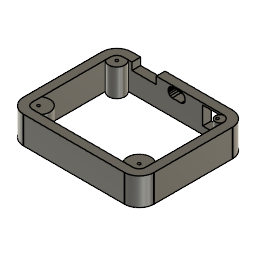
spelarö (Autodesk Fusion 360 design; units mm, degrees)
description: KiCad electronic assembly
part number: spelar_ 1
part number: KEY-SMD_6P-L10.2-W10.2-H10.0-LS11.7-P6.5
part number: C145910
part number: plate and holes
part number: circle001
part number: circle002
part number: circle003
part number: circle004
part number: border001
part number: border002
part number: ShapeString099
part number: ShapeString100
part number: ShapeString101
part number: ShapeString102
part number: ShapeString103
part number: ShapeString104
part number: silk_upper
part number: cupper_upper
part number: cupper_bottom
part number: mask_bottom
part number: res_silk
part number: res_silk001
part number: res_silk002
part number: res_silk003
part number: res_silk004
part number: res_silk005
part number: cap_silk_up
part number: cap_silk_dwn
part number: cap_silk001
part number: cap_silk_up001
part number: cap_silk_dwn001
part number: cap_silk002
part number: sot23_left
part number: sot23_right
part number: sot23_001
part number: sot23_left001
part number: sot23_right001
part number: sot23_002
part number: u2_silk002
part number: sd_silk001
part number: line_silk001
part number: line_silk002
part number: ShapeString067
part number: ShapeString105
part number: ShapeString106
part number: ShapeString107
part number: ShapeString108
part number: ShapeString109
part number: touch
part number: ShapeString068
part number: ShapeString110
part number: ShapeString111
part number: ShapeString112
part number: ShapeString113
part number: ShapeString114
part number: ShapeString069
part number: ShapeString115
part number: ShapeString116
part number: ShapeString117
part number: ShapeString118
part number: ShapeString070
part number: ShapeString119
part number: ShapeString120
part number: ShapeString121
part number: ShapeString122
part number: ShapeString123
part number: ShapeString071
part number: ShapeString124
part number: ShapeString125
part number: ShapeString126
part number: ShapeString127
part number: ShapeString073
part number: ShapeString128
part number: ShapeString129
part number: ShapeString130
part number: ShapeString131
part number: ShapeString132
part number: ShapeString072
part number: ShapeString133
part number: ShapeString134
part number: ShapeString135
part number: ShapeString136
part number: ShapeString137
part number: ShapeString138
part number: ShapeString139
part number: ShapeString140
part number: ShapeString141
part number: ShapeString074
part number: ShapeString142
part number: ShapeString143
part number: ShapeString144
part number: ShapeString075
part number: ShapeString145
part number: ShapeString146
part number: ShapeString147
part number: ShapeString076
part number: ShapeString148
part number: ShapeString149
part number: ShapeString150
part number: ShapeString151
part number: ShapeString152
part number: ShapeString153
part number: ShapeString154
part number: ShapeString155
part number: ShapeString156
part number: ShapeString077
part number: ShapeString157
part number: ShapeString158
part number: ShapeString078
part number: ShapeString159
part number: ShapeString160
part number: ShapeString161
part number: ShapeString162
part number: ShapeString163
part number: ShapeString079
part number: ShapeString164
part number: ShapeString165
part number: ShapeString080
part number: ShapeString166
part number: ShapeString167
part number: ShapeString168
part number: ShapeString081
part number: ShapeString169
part number: ShapeString170
part number: ShapeString171
part number: ShapeString082
part number: ShapeString172
part number: ShapeString173
part number: ShapeString174
part number: ShapeString175
part number: ShapeString176
part number: ShapeString177
part number: ShapeString083
part number: ShapeString178
part number: ShapeString179
part number: ShapeString180
part number: ShapeString181
part number: ShapeString182
part number: ShapeString183
part number: ShapeString184
part number: ShapeString084
part number: ShapeString185
part number: ShapeString186
part number: ShapeString187
part number: ShapeString188
part number: ShapeString189
part number: ShapeString190
part number: ShapeString191
part number: ShapeString085
part number: ShapeString192
part number: ShapeString193
part number: ShapeString194
part number: ShapeString195
part number: ShapeString196
part number: ShapeString086
part number: ShapeString197
part number: ShapeString198
part number: ShapeString199
part number: ShapeString200
part number: ShapeString201
part number: ShapeString202
part number: ShapeString203
part number: ShapeString204
part number: ShapeString205
part number: ShapeString206
part number: ShapeString207
part number: ShapeString208
part number: ShapeString209
part number: ShapeString210
part number: ShapeString211
part number: ShapeString212
part number: ShapeString213
part number: ShapeString214
part number: ShapeString215
part number: ShapeString216
part number: ShapeString217
part number: ShapeString218
part number: ShapeString219
part number: ShapeString220
part number: ShapeString221
part number: ShapeString222
part number: ShapeString087
part number: ShapeString223
part number: ShapeString224
part number: ShapeString088
part number: ShapeString225
part number: ShapeString226
part number: ShapeString089
part number: ShapeString227
part number: ShapeString228
part number: ShapeString090
part number: ShapeString229
part number: ShapeString230
part number: ShapeString091
part number: ShapeString231
part number: ShapeString232
part number: ShapeString092
part number: ShapeString233
part number: ShapeString234
part number: ShapeString093
part number: ShapeString235
part number: ShapeString236
part number: ShapeString094
part number: ShapeString237
part number: ShapeString238
part number: ShapeString095
part number: ShapeString239
part number: ShapeString240
part number: ShapeString096
part number: ShapeString241
part number: ShapeString242
part number: ShapeString097
part number: ShapeString243
part number: ShapeString244
part number: ShapeString098
part number: ShapeString245
part number: ShapeString246
part number: text
part number: j_silk006
part number: silk_bottom
part number: contact01
part number: contact02
part number: contact03
part number: contact04
part number: contact05
part number: contact06
part number: contact07
part number: contact08
part number: frame001
part number: contact09
part number: cover
part number: contact11
part number: contact10
part number: SD slot
part number: TSSOP16_001
part number: TSSOP16_002
part number: TSSOP16_003
part number: TSSOP16_004
part number: TSSOP16_005
part number: TSSOP16_006
part number: TSSOP16_007
part number: TSSOP16_008
part number: TSSOP16_009
part number: ShapeString066
part number: ShapeString247
part number: ShapeString248
part number: ShapeString249
part number: ShapeString250
part number: ShapeString251
part number: ShapeString252
part number: ShapeString253
part number: TSSOP16_010
part number: body
part number: contact1
part number: contact2
part number: label
part number: ShapeString001
part number: ShapeString254
part number: ShapeString255
part number: ShapeString256
part number: Part010
part number: SMD_resistor001
part number: body003
part number: contact016
part number: contact017
part number: label001
part number: ShapeString002
part number: ShapeString257
part number: ShapeString258
part number: ShapeString259
part number: Part013
part number: SMD_resistor002
part number: body004
part number: contact018
part number: contact019
part number: label002
part number: ShapeString003
part number: ShapeString260
part number: ShapeString261
part number: ShapeString262
part number: Part015
part number: SMD_resistor003
part number: body005
part number: contact020
part number: contact021
part number: label003
part number: ShapeString004
part number: ShapeString263
part number: ShapeString264
part number: ShapeString265
part number: Part017
part number: SMD_resistor004
part number: body006
part number: contact022
part number: contact023
part number: label004
part number: ShapeString005
part number: ShapeString266
part number: ShapeString267
part number: ShapeString268
part number: Part019
part number: SMD_resistor005
part number: body007
part number: contact024
part number: contact025
part number: label005
part number: ShapeString006
part number: ShapeString269
part number: ShapeString270
part number: ShapeString271
part number: Part021
part number: SMD_resistor006
part number: body008
part number: contact026
part number: contact027
part number: SMD_cap001
part number: body002
part number: contact014
part number: contact015
part number: SMD_cap002
part number: ShapeString064
part number: ShapeString272
part number: ShapeString273
part number: ShapeString274
part number: Pin036
part number: Pin035
part number: Pin1
part number: Case
part number: SOT23
part number: ShapeString065
part number: ShapeString275
part number: ShapeString276
part number: ShapeString277
part number: ShapeString278
part number: Pin039
part number: Pin038
part number: Pin037
part number: Case001
part number: SOT23-1
part number: parts
part number: Frame
part number: Pin01
part number: Pin002
part number: Pin003
part number: Pin004
part number: Pin005
part number: Pin006
part number: Pin007
part number: Pin008
part number: Pin009
part number: Pin010
part number: Pin011
part number: Pin012
part number: Pin013
part number: Pin014
part number: pls-14
part number: components
part number: mask_upper
part number: Board
part number: frame
part number: metal bandage
part number: light_shelf
part number: main_shelf
part number: tft_cable
part number: tft_matrix
part number: tft_board
part number: tft
part number: screen_film
part number: screen_glass
part number: screen
part number: Display
part number: touch_routs
part number: touch_protect
part number: touch_cable_contacts
part number: touch_cable_film
part number: touch_cable
part number: Touchscreen
part number: Display and Touchscreen
part number: 2.8''LCD_MSP2807
part number: LCD_MSP2807_fusion
part number: VS-1213-67-160GF
part number: C_1206_3216Metric
part number: TF-SMD_TF-012
part number: ESP32 S3 SUPERMINI
part number: ESP32-S3-ZERO
part number: FCR684205R ORJ5
part number: 4654_FCR684205T%20OTJ5
part number: spelarÃ¶_copper
part number: spelarÃ¶_pad
part number: spelarÃ¶_via
part number: spelarÃ¶_silkscreen
part number: spelarÃ¶_soldermask
part number: spelarÃ¶_PCB
Autodesk Fusion 360 part; units mm, degrees
(part 1 of 5)
sketch "Sketch1" plane through (0, 0, 1.56) normal (0, 0, 1) x (-1, 0, 0)
  arc A0 (-129.3118, 35.1924) -> (-124.5324, 39.9718) centre (-129.53, 40.19) ccw
  line L0 (-124.5324, 39.9718) -> (-124.53, 40.19)
  line L1 (-124.53, 40.19) -> (-124.53, 102.8)
  line L2 (-124.53, 102.8) -> (-124.5323, 103.0182)
  arc A1 (-124.5323, 103.0182) -> (-129.3118, 107.7977) centre (-129.53, 102.8) ccw
  line L3 (-129.3118, 107.7977) -> (-129.53, 107.8)
  line L4 (-129.53, 107.8) -> (-210.09, 107.8)
  line L5 (-210.09, 107.8) -> (-210.3082, 107.7977)
  arc A2 (-210.3082, 107.7977) -> (-215.0877, 103.0182) centre (-210.09, 102.8) ccw
  line L6 (-215.0877, 103.0182) -> (-215.09, 102.8)
  line L7 (-215.09, 102.8) -> (-215.09, 40.19)
  line L8 (-215.09, 40.19) -> (-215.0876, 39.9718)
  arc A3 (-215.0876, 39.9718) -> (-210.3082, 35.1924) centre (-210.09, 40.19) ccw
  line L9 (-210.3082, 35.1924) -> (-210.09, 35.19)
  line L10 (-210.09, 35.19) -> (-129.53, 35.19)
  line L11 (-129.53, 35.19) -> (-129.3118, 35.1924)
  circle A4 centre (-129.53, 102.8) radius 2.2
  circle A5 centre (-210.09, 102.8) radius 2.2
  line L12 (-153, 103.32) -> (-153, 104.72)
  line L13 (-153, 104.72) -> (-151, 104.72)
  line L14 (-151, 104.72) -> (-151, 103.32)
  line L15 (-151, 103.32) -> (-153, 103.32)
  line L16 (-164.46, 103.32) -> (-164.46, 104.72)
  line L17 (-164.46, 104.72) -> (-162.46, 104.72)
  line L18 (-162.46, 104.72) -> (-162.46, 103.32)
  line L19 (-162.46, 103.32) -> (-164.46, 103.32)
  circle A6 centre (-172, 103.08) radius 1.077
  circle A7 centre (-184.5, 103.08) radius 1.077
  line L20 (-153, 100.52) -> (-153, 101.92)
  line L21 (-153, 101.92) -> (-151, 101.92)
  line L22 (-151, 101.92) -> (-151, 100.52)
  line L23 (-151, 100.52) -> (-153, 100.52)
  line L24 (-164.46, 100.52) -> (-164.46, 101.92)
  line L25 (-164.46, 101.92) -> (-162.46, 101.92)
  line L26 (-162.46, 101.92) -> (-162.46, 100.52)
  line L27 (-162.46, 100.52) -> (-164.46, 100.52)
  arc A8 (-173.077, 97.105) -> (-172.975, 97.003) centre (-172.975, 97.105) ccw
  line L28 (-173.077, 97.105) -> (-173.077, 99.055)
  arc A9 (-172.975, 99.157) -> (-173.077, 99.055) centre (-172.975, 99.055) ccw
  line L29 (-172.975, 99.157) -> (-171.025, 99.157)
  arc A10 (-170.923, 99.055) -> (-171.025, 99.157) centre (-171.025, 99.055) ccw
  line L30 (-170.923, 99.055) -> (-170.923, 97.105)
  arc A11 (-171.025, 97.003) -> (-170.923, 97.105) centre (-171.025, 97.105) ccw
  line L31 (-171.025, 97.003) -> (-172.975, 97.003)
  circle A12 centre (-184.5, 98.08) radius 1.077
  line L32 (-153, 96.82) -> (-153, 98.22)
  line L33 (-153, 98.22) -> (-151, 98.22)
  line L34 (-151, 98.22) -> (-151, 96.82)
  line L35 (-151, 96.82) -> (-153, 96.82)
  line L36 (-164.46, 96.82) -> (-164.46, 98.22)
  line L37 (-164.46, 98.22) -> (-162.46, 98.22)
  line L38 (-162.46, 98.22) -> (-162.46, 96.82)
  line L39 (-162.46, 96.82) -> (-164.46, 96.82)
  line L40 (-212.43, 77.21) -> (-212.43, 78.91)
  line L41 (-212.43, 78.91) -> (-210.73, 78.91)
  line L42 (-210.73, 78.91) -> (-210.73, 77.21)
  line L43 (-210.73, 77.21) -> (-212.43, 77.21)
  circle A13 centre (-211.58, 75.52) radius 0.85
  circle A14 centre (-211.58, 72.98) radius 0.85
  circle A15 centre (-211.58, 70.44) radius 0.85
  circle A16 centre (-211.58, 67.9) radius 0.85
  circle A17 centre (-211.58, 65.36) radius 0.85
  circle A18 centre (-211.58, 62.82) radius 0.85
  circle A19 centre (-211.58, 60.28) radius 0.85
  circle A20 centre (-211.58, 57.74) radius 0.85
  circle A21 centre (-211.58, 55.2) radius 0.85
  circle A22 centre (-211.58, 52.66) radius 0.85
  circle A23 centre (-211.58, 50.12) radius 0.85
  circle A24 centre (-211.58, 47.58) radius 0.85
  circle A25 centre (-196.89, 46.1501) radius 0.6604
  circle A26 centre (-199.43, 46.1501) radius 0.6604
  circle A27 centre (-201.97, 46.1501) radius 0.6604
  circle A28 centre (-211.58, 45.04) radius 0.85
  circle A29 centre (-129.53, 40.19) radius 2.2
  circle A30 centre (-210.09, 40.19) radius 2.2
  arc A31 (-222.0862, 39.8056) -> (-210.4744, 28.1938) centre (-210.09, 40.19) ccw
  line L44 (-210.4744, 28.1938) -> (-210.1282, 28.19)
  line L45 (-210.1282, 28.19) -> (-129.4918, 28.19)
  line L46 (-129.4918, 28.19) -> (-129.1456, 28.1938)
  arc A32 (-129.1456, 28.1938) -> (-117.5338, 39.8056) centre (-129.53, 40.19) ccw
  line L47 (-117.5338, 39.8056) -> (-117.53, 40.1518)
  line L48 (-117.53, 40.1518) -> (-117.53, 102.8371)
  line L49 (-117.53, 102.8371) -> (-117.5337, 103.1831)
  arc A33 (-117.5337, 103.1831) -> (-129.1469, 114.7963) centre (-129.53, 102.8) ccw
  line L50 (-129.1469, 114.7963) -> (-129.4929, 114.8)
  line L51 (-129.4929, 114.8) -> (-210.1271, 114.8)
  line L52 (-210.1271, 114.8) -> (-210.4731, 114.7963)
  arc A34 (-210.4731, 114.7963) -> (-222.0863, 103.1831) centre (-210.09, 102.8) ccw
  line L53 (-222.0863, 103.1831) -> (-222.09, 102.8371)
  line L54 (-222.09, 102.8371) -> (-222.09, 40.1518)
  line L55 (-222.09, 40.1518) -> (-222.0862, 39.8056)
  dimension "d1" = 7
extrude "Extrude1" add sketch "Sketch1" against normal blind 22 contours A31 L44 L45 L46 A32 L47 L48 L49 A33 L50 L51 L52 A34 L53 L54 L55
sketch "Sketch2" plane through (0, -28.19, 0) normal (0, 1, 0) x (-1, 0, 0)
  line L0 (-129.4918, 1.56) -> (-210.1282, 1.56)
  line L1 (-210.1282, 1.56) -> (-210.1282, -20.44)
  line L2 (-210.1282, -20.44) -> (-129.4918, -20.44)
  line L3 (-129.4918, -20.44) -> (-129.4918, 1.56)
  line L4 (-153.8, -0.2) -> (-139, -0.2)
  line L5 (-139, -0.2) -> (-139, -2)
  line L6 (-139, -2) -> (-153.8, -2)
  line L7 (-153.8, -2) -> (-153.8, -0.2)
  line L8 (-156.1178, -4.3178) -> (-156.1178, 2.1178)
  line L9 (-156.1178, 2.1178) -> (-136.6822, 2.1178)
  line L10 (-136.6822, 2.1178) -> (-136.6822, -4.3178)
  line L11 (-136.6822, -4.3178) -> (-156.1178, -4.3178)
  dimension "d4" = -2.3178
  constraint horizontal L4
  constraint vertical L5
  constraint horizontal L6
  constraint vertical L7
extrude "Extrude2" cut sketch "Sketch2" against normal blind 7 contours L0 L8 L10 L11 | L4 L5 L6 L7
sketch "Sketch3" plane through (0, -28.19, 0) normal (0, 1, 0) x (-1, 0, 0)
  line L0 (-136.6822, 1.56) -> (-136.6822, -4.3178)
  line L1 (-136.6822, -4.3178) -> (-156.1178, -4.3178)
  line L2 (-156.1178, -4.3178) -> (-156.1178, 1.56)
  line L3 (-156.1178, 1.56) -> (-210.1282, 1.56)
  line L4 (-210.1282, 1.56) -> (-210.1282, -20.44)
  line L5 (-210.1282, -20.44) -> (-129.4918, -20.44)
  line L6 (-129.4918, -20.44) -> (-129.4918, 1.56)
  line L7 (-129.4918, 1.56) -> (-136.6822, 1.56)
  line L8 (-175.65, -1.85) -> (-169.25, -1.85)
  line L9 (-169.25, -1.85) -> (-168.6525, -2.0383)
  line L10 (-168.6525, -2.0383) -> (-168.3, -2.4)
  line L11 (-168.3, -2.4) -> (-168.1, -2.7)
  line L12 (-168.1, -2.7) -> (-168.0543, -2.9985)
  line L13 (-168.0543, -2.9985) -> (-168.0543, -3.7)
  line L14 (-168.0543, -3.7) -> (-168.1, -4.044)
  line L15 (-168.1, -4.044) -> (-168.2705, -4.3456)
  line L16 (-168.2705, -4.3456) -> (-168.5369, -4.6523)
  line L17 (-168.5369, -4.6523) -> (-169.2457, -4.8986)
  line L18 (-169.2457, -4.8986) -> (-175.7, -4.8986)
  line L19 (-175.7, -4.8986) -> (-176.2708, -4.724)
  line L20 (-176.2708, -4.724) -> (-176.6, -4.35)
  line L21 (-176.6, -4.35) -> (-176.8, -4)
  line L22 (-176.8, -4) -> (-176.85, -3.7)
  line L23 (-176.85, -3.7) -> (-176.8, -2.9)
  line L24 (-176.8, -2.9) -> (-176.6204, -2.414)
  line L25 (-176.6204, -2.414) -> (-176.1201, -1.9736)
  line L26 (-176.1201, -1.9736) -> (-175.65, -1.85)
  line L27 (-179.0982, -2.4144) -> (-178.5967, -1.0576)
  line L28 (-178.5967, -1.0576) -> (-177.2431, 0.1341)
  line L29 (-177.2431, 0.1341) -> (-175.9505, 0.474)
  line L30 (-175.9505, 0.474) -> (-168.8924, 0.474)
  line L31 (-168.8924, 0.474) -> (-167.3963, 0.0024)
  line L32 (-167.3963, 0.0024) -> (-166.4856, -0.9319)
  line L33 (-166.4856, -0.9319) -> (-165.8806, -1.8394)
  line L34 (-165.8806, -1.8394) -> (-165.7303, -2.8217)
  line L35 (-165.7303, -2.8217) -> (-165.7303, -3.8535)
  line L36 (-165.7303, -3.8535) -> (-165.8554, -4.7959)
  line L37 (-165.8554, -4.7959) -> (-166.3626, -5.6931)
  line L38 (-166.3626, -5.6931) -> (-167.1889, -6.6442)
  line L39 (-167.1889, -6.6442) -> (-168.8534, -7.2226)
  line L40 (-168.8534, -7.2226) -> (-176.0475, -7.2226)
  line L41 (-176.0475, -7.2226) -> (-177.5801, -6.7537)
  line L42 (-177.5801, -6.7537) -> (-178.5005, -5.7083)
  line L43 (-178.5005, -5.7083) -> (-179.0241, -4.7921)
  line L44 (-179.0241, -4.7921) -> (-179.1861, -3.8201)
  line L45 (-179.1861, -3.8201) -> (-179.0982, -2.4144)
  dimension "d7" = -2.324
  constraint horizontal L8
  constraint perpendicular L8 L13
  constraint parallel L8 L18
  constraint perpendicular L20 L25
extrude "Extrude3" cut sketch "Sketch3" against normal blind 7 contours L8 L9 L10 L11 L12 L13 L14 L15 L16 L17 L18 L19 L20 L21 L22 L23 L24 L25 L26 | L27 L28 L29 L30 L31 L32 L33 L34 L35 L36 L37 L38 L39 L40 L41 L42 L43 L44 L45
sketch "Sketch4" plane through (0, -28.19, 0) normal (0, 1, 0) x (-1, 0, 0)
  line L0 (-178.5005, -5.7083) -> (-179.0241, -4.7921)
  line L1 (-179.0241, -4.7921) -> (-179.1861, -3.8201)
  line L2 (-179.1861, -3.8201) -> (-179.0982, -2.4144)
  line L3 (-179.0982, -2.4144) -> (-178.5967, -1.0576)
  line L4 (-178.5967, -1.0576) -> (-177.2431, 0.1341)
  line L5 (-177.2431, 0.1341) -> (-175.9505, 0.474)
  line L6 (-175.9505, 0.474) -> (-168.8924, 0.474)
  line L7 (-168.8924, 0.474) -> (-167.3963, 0.0024)
  line L8 (-167.3963, 0.0024) -> (-166.4856, -0.9319)
  line L9 (-166.4856, -0.9319) -> (-165.8806, -1.8394)
  line L10 (-165.8806, -1.8394) -> (-165.7303, -2.8217)
  line L11 (-165.7303, -2.8217) -> (-165.7303, -3.8535)
  line L12 (-165.7303, -3.8535) -> (-165.8554, -4.7959)
  line L13 (-165.8554, -4.7959) -> (-166.3626, -5.6931)
  line L14 (-166.3626, -5.6931) -> (-167.1889, -6.6442)
  line L15 (-167.1889, -6.6442) -> (-168.8534, -7.2226)
  line L16 (-168.8534, -7.2226) -> (-176.0475, -7.2226)
  line L17 (-176.0475, -7.2226) -> (-177.5801, -6.7537)
  line L18 (-177.5801, -6.7537) -> (-178.5005, -5.7083)
  line L19 (-136.6822, 1.56) -> (-136.6822, -4.3178)
  line L20 (-136.6822, -4.3178) -> (-156.1178, -4.3178)
  line L21 (-156.1178, -4.3178) -> (-156.1178, 1.56)
  line L22 (-156.1178, 1.56) -> (-210.1282, 1.56)
  line L23 (-210.1282, 1.56) -> (-210.1282, -20.44)
  line L24 (-210.1282, -20.44) -> (-129.4918, -20.44)
  line L25 (-129.4918, -20.44) -> (-129.4918, 1.56)
  line L26 (-129.4918, 1.56) -> (-136.6822, 1.56)
  line L27 (-196.1, -11.6) -> (-202.8938, -11.6)
  line L28 (-202.8938, -11.6) -> (-202.8938, -2.8236)
  line L29 (-202.8938, -2.8236) -> (-196.1, -2.8236)
  line L30 (-196.1, -2.8236) -> (-196.1, -11.6)
  line L31 (-193.7671, -0.4907) -> (-193.7671, -13.9329)
  line L32 (-193.7671, -13.9329) -> (-205.2267, -13.9329)
  line L33 (-205.2267, -13.9329) -> (-205.2267, -0.4907)
  line L34 (-205.2267, -0.4907) -> (-193.7671, -0.4907)
  dimension "d10" = -2.3329
  constraint horizontal L27
  constraint vertical L28
  constraint horizontal L29
  constraint vertical L30
extrude "Extrude4" cut sketch "Sketch4" against normal blind 7.5 contours L27 L28 L29 L30 | L31 L32 L33 L34
sketch "Sketch5" plane through (0, 0, 1.56) normal (0, 0, 1) x (-1, 0, 0)
  arc A0 (-129.3118, 35.1924) -> (-124.5324, 39.9718) centre (-129.53, 40.19) ccw
  line L0 (-124.5324, 39.9718) -> (-124.53, 40.19)
  line L1 (-124.53, 40.19) -> (-124.53, 102.8)
  line L2 (-124.53, 102.8) -> (-124.5323, 103.0182)
  arc A1 (-124.5323, 103.0182) -> (-129.3118, 107.7977) centre (-129.53, 102.8) ccw
  line L3 (-129.3118, 107.7977) -> (-129.53, 107.8)
  line L4 (-129.53, 107.8) -> (-210.09, 107.8)
  line L5 (-210.09, 107.8) -> (-210.3082, 107.7977)
  arc A2 (-210.3082, 107.7977) -> (-215.0877, 103.0182) centre (-210.09, 102.8) ccw
  line L6 (-215.0877, 103.0182) -> (-215.09, 102.8)
  line L7 (-215.09, 102.8) -> (-215.09, 40.19)
  line L8 (-215.09, 40.19) -> (-215.0876, 39.9718)
  arc A3 (-215.0876, 39.9718) -> (-210.3082, 35.1924) centre (-210.09, 40.19) ccw
  line L9 (-210.3082, 35.1924) -> (-210.09, 35.19)
  line L10 (-210.09, 35.19) -> (-129.53, 35.19)
  line L11 (-129.53, 35.19) -> (-129.3118, 35.1924)
  circle A4 centre (-129.53, 102.8) radius 2.2
  circle A5 centre (-210.09, 102.8) radius 2.2
  line L12 (-153, 103.32) -> (-153, 104.72)
  line L13 (-153, 104.72) -> (-151, 104.72)
  line L14 (-151, 104.72) -> (-151, 103.32)
  line L15 (-151, 103.32) -> (-153, 103.32)
  line L16 (-164.46, 103.32) -> (-164.46, 104.72)
  line L17 (-164.46, 104.72) -> (-162.46, 104.72)
  line L18 (-162.46, 104.72) -> (-162.46, 103.32)
  line L19 (-162.46, 103.32) -> (-164.46, 103.32)
  circle A6 centre (-172, 103.08) radius 1.077
  circle A7 centre (-184.5, 103.08) radius 1.077
  line L20 (-153, 100.52) -> (-153, 101.92)
  line L21 (-153, 101.92) -> (-151, 101.92)
  line L22 (-151, 101.92) -> (-151, 100.52)
  line L23 (-151, 100.52) -> (-153, 100.52)
  line L24 (-164.46, 100.52) -> (-164.46, 101.92)
  line L25 (-164.46, 101.92) -> (-162.46, 101.92)
  line L26 (-162.46, 101.92) -> (-162.46, 100.52)
  line L27 (-162.46, 100.52) -> (-164.46, 100.52)
  arc A8 (-173.077, 97.105) -> (-172.975, 97.003) centre (-172.975, 97.105) ccw
  line L28 (-173.077, 97.105) -> (-173.077, 99.055)
  arc A9 (-172.975, 99.157) -> (-173.077, 99.055) centre (-172.975, 99.055) ccw
  line L29 (-172.975, 99.157) -> (-171.025, 99.157)
  arc A10 (-170.923, 99.055) -> (-171.025, 99.157) centre (-171.025, 99.055) ccw
  line L30 (-170.923, 99.055) -> (-170.923, 97.105)
  arc A11 (-171.025, 97.003) -> (-170.923, 97.105) centre (-171.025, 97.105) ccw
  line L31 (-171.025, 97.003) -> (-172.975, 97.003)
  circle A12 centre (-184.5, 98.08) radius 1.077
  line L32 (-153, 96.82) -> (-153, 98.22)
  line L33 (-153, 98.22) -> (-151, 98.22)
  line L34 (-151, 98.22) -> (-151, 96.82)
  line L35 (-151, 96.82) -> (-153, 96.82)
  line L36 (-164.46, 96.82) -> (-164.46, 98.22)
  line L37 (-164.46, 98.22) -> (-162.46, 98.22)
  line L38 (-162.46, 98.22) -> (-162.46, 96.82)
  line L39 (-162.46, 96.82) -> (-164.46, 96.82)
  line L40 (-212.43, 77.21) -> (-212.43, 78.91)
  line L41 (-212.43, 78.91) -> (-210.73, 78.91)
  line L42 (-210.73, 78.91) -> (-210.73, 77.21)
  line L43 (-210.73, 77.21) -> (-212.43, 77.21)
  circle A13 centre (-211.58, 75.52) radius 0.85
  circle A14 centre (-211.58, 72.98) radius 0.85
  circle A15 centre (-211.58, 70.44) radius 0.85
  circle A16 centre (-211.58, 67.9) radius 0.85
  circle A17 centre (-211.58, 65.36) radius 0.85
  circle A18 centre (-211.58, 62.82) radius 0.85
  circle A19 centre (-211.58, 60.28) radius 0.85
  circle A20 centre (-211.58, 57.74) radius 0.85
  circle A21 centre (-211.58, 55.2) radius 0.85
  circle A22 centre (-211.58, 52.66) radius 0.85
  circle A23 centre (-211.58, 50.12) radius 0.85
  circle A24 centre (-211.58, 47.58) radius 0.85
  circle A25 centre (-196.89, 46.1501) radius 0.6604
  circle A26 centre (-199.43, 46.1501) radius 0.6604
  circle A27 centre (-201.97, 46.1501) radius 0.6604
  circle A28 centre (-211.58, 45.04) radius 0.85
  circle A29 centre (-129.53, 40.19) radius 2.2
  circle A30 centre (-210.09, 40.19) radius 2.2
  circle A31 centre (-210.09, 102.8006) radius 2.1994
  circle A32 centre (-210.09, 102.8006) radius 1.0859
  dimension "d26" = -1.1134
  constraint tangent A5 A31
sketch "Sketch6" plane through (0, 0, -0.05) normal (0, 0, -1) x (1, 0, 0)
  arc A0 (124.5324, 39.9718) -> (129.3118, 35.1924) centre (129.53, 40.19) ccw
  line L0 (129.3118, 35.1924) -> (129.53, 35.19)
  line L1 (129.53, 35.19) -> (210.09, 35.19)
  line L2 (210.09, 35.19) -> (210.3082, 35.1924)
  arc A1 (210.3082, 35.1924) -> (215.0876, 39.9718) centre (210.09, 40.19) ccw
  line L3 (215.0876, 39.9718) -> (215.09, 40.19)
  line L4 (215.09, 40.19) -> (215.09, 102.8)
  line L5 (215.09, 102.8) -> (215.0877, 103.0182)
  arc A2 (215.0877, 103.0182) -> (210.3082, 107.7977) centre (210.09, 102.8) ccw
  line L6 (210.3082, 107.7977) -> (210.09, 107.8)
  line L7 (210.09, 107.8) -> (129.53, 107.8)
  line L8 (129.53, 107.8) -> (129.3118, 107.7977)
  arc A3 (129.3118, 107.7977) -> (124.5323, 103.0182) centre (129.53, 102.8) ccw
  line L9 (124.5323, 103.0182) -> (124.53, 102.8)
  line L10 (124.53, 102.8) -> (124.53, 40.19)
  line L11 (124.53, 40.19) -> (124.5324, 39.9718)
  circle A4 centre (172, 103.08) radius 1.077
  circle A5 centre (184.5, 103.08) radius 1.077
  circle A6 centre (129.53, 102.8) radius 1.3
  circle A7 centre (210.09, 102.8) radius 1.3
  arc A8 (172.975, 97.003) -> (173.077, 97.105) centre (172.975, 97.105) ccw
  line L12 (172.975, 97.003) -> (171.025, 97.003)
  arc A9 (170.923, 97.105) -> (171.025, 97.003) centre (171.025, 97.105) ccw
  line L13 (170.923, 97.105) -> (170.923, 99.055)
  arc A10 (171.025, 99.157) -> (170.923, 99.055) centre (171.025, 99.055) ccw
  line L14 (171.025, 99.157) -> (172.975, 99.157)
  arc A11 (173.077, 99.055) -> (172.975, 99.157) centre (172.975, 99.055) ccw
  line L15 (173.077, 99.055) -> (173.077, 97.105)
  circle A12 centre (184.5, 98.08) radius 1.077
  line L16 (212.43, 78.91) -> (212.43, 77.21)
  line L17 (212.43, 77.21) -> (210.73, 77.21)
  line L18 (210.73, 77.21) -> (210.73, 78.91)
  line L19 (210.73, 78.91) -> (212.43, 78.91)
  circle A13 centre (211.58, 75.52) radius 0.85
  circle A14 centre (211.58, 72.98) radius 0.85
  circle A15 centre (211.58, 70.44) radius 0.85
  circle A16 centre (211.58, 67.9) radius 0.85
  circle A17 centre (211.58, 65.36) radius 0.85
  circle A18 centre (211.58, 62.82) radius 0.85
  circle A19 centre (211.58, 60.28) radius 0.85
  arc A20 (164.6391, 57.504) -> (164.7411, 57.606) centre (164.6391, 57.606) ccw
  line L20 (164.6391, 57.504) -> (162.6391, 57.504)
  arc A21 (162.5371, 57.606) -> (162.6391, 57.504) centre (162.6391, 57.606) ccw
  line L21 (162.5371, 57.606) -> (162.5371, 59.114)
  arc A22 (162.6391, 59.216) -> (162.5371, 59.114) centre (162.6391, 59.114) ccw
  line L22 (162.6391, 59.216) -> (164.6391, 59.216)
  arc A23 (164.7411, 59.114) -> (164.6391, 59.216) centre (164.6391, 59.114) ccw
  line L23 (164.7411, 59.114) -> (164.7411, 57.606)
  arc A24 (182.0197, 57.504) -> (182.1217, 57.606) centre (182.0197, 57.606) ccw
  line L24 (182.0197, 57.504) -> (180.0197, 57.504)
  arc A25 (179.9177, 57.606) -> (180.0197, 57.504) centre (180.0197, 57.606) ccw
  line L25 (179.9177, 57.606) -> (179.9177, 59.114)
  arc A26 (180.0197, 59.216) -> (179.9177, 59.114) centre (180.0197, 59.114) ccw
  line L26 (180.0197, 59.216) -> (182.0197, 59.216)
  arc A27 (182.1217, 59.114) -> (182.0197, 59.216) centre (182.0197, 59.114) ccw
  line L27 (182.1217, 59.114) -> (182.1217, 57.606)
  circle A28 centre (211.58, 57.74) radius 0.85
  arc A29 (164.6322, 54.964) -> (164.7342, 55.066) centre (164.6322, 55.066) ccw
  line L28 (164.6322, 54.964) -> (162.6322, 54.964)
  arc A30 (162.5302, 55.066) -> (162.6322, 54.964) centre (162.6322, 55.066) ccw
  line L29 (162.5302, 55.066) -> (162.5302, 56.574)
  arc A31 (162.6322, 56.676) -> (162.5302, 56.574) centre (162.6322, 56.574) ccw
  line L30 (162.6322, 56.676) -> (164.6322, 56.676)
  arc A32 (164.7342, 56.574) -> (164.6322, 56.676) centre (164.6322, 56.574) ccw
  line L31 (164.7342, 56.574) -> (164.7342, 55.066)
  arc A33 (182.0197, 54.964) -> (182.1217, 55.066) centre (182.0197, 55.066) ccw
  line L32 (182.0197, 54.964) -> (180.0197, 54.964)
  arc A34 (179.9177, 55.066) -> (180.0197, 54.964) centre (180.0197, 55.066) ccw
  line L33 (179.9177, 55.066) -> (179.9177, 56.574)
  arc A35 (180.0197, 56.676) -> (179.9177, 56.574) centre (180.0197, 56.574) ccw
  line L34 (180.0197, 56.676) -> (182.0197, 56.676)
  arc A36 (182.1217, 56.574) -> (182.0197, 56.676) centre (182.0197, 56.574) ccw
  line L35 (182.1217, 56.574) -> (182.1217, 55.066)
  circle A37 centre (211.58, 55.2) radius 0.85
  arc A38 (199.24, 52.73) -> (199.49, 52.98) centre (199.24, 52.98) ccw
  line L36 (199.24, 52.73) -> (198.59, 52.73)
  arc A39 (198.34, 52.98) -> (198.59, 52.73) centre (198.59, 52.98) ccw
  line L37 (198.34, 52.98) -> (198.34, 54.28)
  arc A40 (198.59, 54.53) -> (198.34, 54.28) centre (198.59, 54.28) ccw
  line L38 (198.59, 54.53) -> (199.24, 54.53)
  arc A41 (199.49, 54.28) -> (199.24, 54.53) centre (199.24, 54.28) ccw
  line L39 (199.49, 54.28) -> (199.49, 52.98)
  arc A42 (202.19, 52.73) -> (202.44, 52.98) centre (202.19, 52.98) ccw
  line L40 (202.19, 52.73) -> (201.54, 52.73)
  arc A43 (201.29, 52.98) -> (201.54, 52.73) centre (201.54, 52.98) ccw
  line L41 (201.29, 52.98) -> (201.29, 54.28)
  arc A44 (201.54, 54.53) -> (201.29, 54.28) centre (201.54, 54.28) ccw
  line L42 (201.54, 54.53) -> (202.19, 54.53)
  arc A45 (202.44, 54.28) -> (202.19, 54.53) centre (202.19, 54.28) ccw
  line L43 (202.44, 54.28) -> (202.44, 52.98)
  arc A46 (164.6322, 52.424) -> (164.7342, 52.526) centre (164.6322, 52.526) ccw
  line L44 (164.6322, 52.424) -> (162.6322, 52.424)
  arc A47 (162.5302, 52.526) -> (162.6322, 52.424) centre (162.6322, 52.526) ccw
  line L45 (162.5302, 52.526) -> (162.5302, 54.034)
  arc A48 (162.6322, 54.136) -> (162.5302, 54.034) centre (162.6322, 54.034) ccw
  line L46 (162.6322, 54.136) -> (164.6322, 54.136)
  arc A49 (164.7342, 54.034) -> (164.6322, 54.136) centre (164.6322, 54.034) ccw
  line L47 (164.7342, 54.034) -> (164.7342, 52.526)
  arc A50 (182.0197, 52.424) -> (182.1217, 52.526) centre (182.0197, 52.526) ccw
  line L48 (182.0197, 52.424) -> (180.0197, 52.424)
  arc A51 (179.9177, 52.526) -> (180.0197, 52.424) centre (180.0197, 52.526) ccw
  line L49 (179.9177, 52.526) -> (179.9177, 54.034)
  arc A52 (180.0197, 54.136) -> (179.9177, 54.034) centre (180.0197, 54.034) ccw
  line L50 (180.0197, 54.136) -> (182.0197, 54.136)
  arc A53 (182.1217, 54.034) -> (182.0197, 54.136) centre (182.0197, 54.034) ccw
  line L51 (182.1217, 54.034) -> (182.1217, 52.526)
  circle A54 centre (211.58, 52.66) radius 0.85
  arc A55 (164.6322, 49.884) -> (164.7342, 49.986) centre (164.6322, 49.986) ccw
  line L52 (164.6322, 49.884) -> (162.6322, 49.884)
  arc A56 (162.5302, 49.986) -> (162.6322, 49.884) centre (162.6322, 49.986) ccw
  line L53 (162.5302, 49.986) -> (162.5302, 51.494)
  arc A57 (162.6322, 51.596) -> (162.5302, 51.494) centre (162.6322, 51.494) ccw
  line L54 (162.6322, 51.596) -> (164.6322, 51.596)
  arc A58 (164.7342, 51.494) -> (164.6322, 51.596) centre (164.6322, 51.494) ccw
  line L55 (164.7342, 51.494) -> (164.7342, 49.986)
  arc A59 (182.0197, 49.884) -> (182.1217, 49.986) centre (182.0197, 49.986) ccw
  line L56 (182.0197, 49.884) -> (180.0197, 49.884)
  arc A60 (179.9177, 49.986) -> (180.0197, 49.884) centre (180.0197, 49.986) ccw
  line L57 (179.9177, 49.986) -> (179.9177, 51.494)
  arc A61 (180.0197, 51.596) -> (179.9177, 51.494) centre (180.0197, 51.494) ccw
  line L58 (180.0197, 51.596) -> (182.0197, 51.596)
  arc A62 (182.1217, 51.494) -> (182.0197, 51.596) centre (182.0197, 51.494) ccw
  line L59 (182.1217, 51.494) -> (182.1217, 49.986)
  line L60 (140.26, 51.04) -> (140.26, 49.44)
  line L61 (140.26, 49.44) -> (139.56, 49.44)
  line L62 (139.56, 49.44) -> (139.56, 51.04)
  line L63 (139.56, 51.04) -> (140.26, 51.04)
  line L64 (141.36, 51.04) -> (141.36, 49.44)
  line L65 (141.36, 49.44) -> (140.66, 49.44)
  line L66 (140.66, 49.44) -> (140.66, 51.04)
  line L67 (140.66, 51.04) -> (141.36, 51.04)
  line L68 (142.46, 51.04) -> (142.46, 49.44)
  line L69 (142.46, 49.44) -> (141.76, 49.44)
  line L70 (141.76, 49.44) -> (141.76, 51.04)
  line L71 (141.76, 51.04) -> (142.46, 51.04)
  line L72 (143.56, 51.04) -> (143.56, 49.44)
  line L73 (143.56, 49.44) -> (142.86, 49.44)
  line L74 (142.86, 49.44) -> (142.86, 51.04)
  line L75 (142.86, 51.04) -> (143.56, 51.04)
  line L76 (144.66, 51.04) -> (144.66, 49.44)
  line L77 (144.66, 49.44) -> (143.96, 49.44)
  line L78 (143.96, 49.44) -> (143.96, 51.04)
  line L79 (143.96, 51.04) -> (144.66, 51.04)
  line L80 (145.76, 51.04) -> (145.76, 49.44)
  line L81 (145.76, 49.44) -> (145.06, 49.44)
  line L82 (145.06, 49.44) -> (145.06, 51.04)
  line L83 (145.06, 51.04) -> (145.76, 51.04)
  line L84 (146.86, 51.04) -> (146.86, 49.44)
  line L85 (146.86, 49.44) -> (146.16, 49.44)
  line L86 (146.16, 49.44) -> (146.16, 51.04)
  line L87 (146.16, 51.04) -> (146.86, 51.04)
  line L88 (147.96, 51.04) -> (147.96, 49.44)
  line L89 (147.96, 49.44) -> (147.26, 49.44)
  line L90 (147.26, 49.44) -> (147.26, 51.04)
  line L91 (147.26, 51.04) -> (147.96, 51.04)
  line L92 (149.06, 51.04) -> (149.06, 49.44)
  line L93 (149.06, 49.44) -> (148.36, 49.44)
  line L94 (148.36, 49.44) -> (148.36, 51.04)
  line L95 (148.36, 51.04) -> (149.06, 51.04)
  circle A63 centre (211.58, 50.12) radius 0.85
  line L96 (139.26, 49.99) -> (139.26, 48.49)
  line L97 (139.26, 48.49) -> (138.06, 48.49)
  line L98 (138.06, 48.49) -> (138.06, 49.99)
  line L99 (138.06, 49.99) -> (139.26, 49.99)
  line L100 (154.11, 49.99) -> (154.11, 48.49)
  line L101 (154.11, 48.49) -> (152.51, 48.49)
  line L102 (152.51, 48.49) -> (152.51, 49.99)
  line L103 (152.51, 49.99) -> (154.11, 49.99)
  arc A64 (164.6322, 47.344) -> (164.7342, 47.446) centre (164.6322, 47.446) ccw
  line L104 (164.6322, 47.344) -> (162.6322, 47.344)
  arc A65 (162.5302, 47.446) -> (162.6322, 47.344) centre (162.6322, 47.446) ccw
  line L105 (162.5302, 47.446) -> (162.5302, 48.954)
  arc A66 (162.6322, 49.056) -> (162.5302, 48.954) centre (162.6322, 48.954) ccw
  line L106 (162.6322, 49.056) -> (164.6322, 49.056)
  arc A67 (164.7342, 48.954) -> (164.6322, 49.056) centre (164.6322, 48.954) ccw
  line L107 (164.7342, 48.954) -> (164.7342, 47.446)
  arc A68 (182.0197, 47.344) -> (182.1217, 47.446) centre (182.0197, 47.446) ccw
  line L108 (182.0197, 47.344) -> (180.0197, 47.344)
  arc A69 (179.9177, 47.446) -> (180.0197, 47.344) centre (180.0197, 47.446) ccw
  line L109 (179.9177, 47.446) -> (179.9177, 48.954)
  arc A70 (180.0197, 49.056) -> (179.9177, 48.954) centre (180.0197, 48.954) ccw
  line L110 (180.0197, 49.056) -> (182.0197, 49.056)
  arc A71 (182.1217, 48.954) -> (182.0197, 49.056) centre (182.0197, 48.954) ccw
  line L111 (182.1217, 48.954) -> (182.1217, 47.446)
  circle A72 centre (211.58, 47.58) radius 0.85
  circle A73 centre (196.89, 46.1501) radius 0.6604
  circle A74 centre (199.43, 46.1501) radius 0.6604
  circle A75 centre (201.97, 46.1501) radius 0.6604
  arc A76 (164.6322, 44.804) -> (164.7342, 44.906) centre (164.6322, 44.906) ccw
  line L112 (164.6322, 44.804) -> (162.6322, 44.804)
  arc A77 (162.5302, 44.906) -> (162.6322, 44.804) centre (162.6322, 44.906) ccw
  line L113 (162.5302, 44.906) -> (162.5302, 46.414)
  arc A78 (162.6322, 46.516) -> (162.5302, 46.414) centre (162.6322, 46.414) ccw
  line L114 (162.6322, 46.516) -> (164.6322, 46.516)
  arc A79 (164.7342, 46.414) -> (164.6322, 46.516) centre (164.6322, 46.414) ccw
  line L115 (164.7342, 46.414) -> (164.7342, 44.906)
  arc A80 (182.0197, 44.804) -> (182.1217, 44.906) centre (182.0197, 44.906) ccw
  line L116 (182.0197, 44.804) -> (180.0197, 44.804)
  arc A81 (179.9177, 44.906) -> (180.0197, 44.804) centre (180.0197, 44.906) ccw
  line L117 (179.9177, 44.906) -> (179.9177, 46.414)
  arc A82 (180.0197, 46.516) -> (179.9177, 46.414) centre (180.0197, 46.414) ccw
  line L118 (180.0197, 46.516) -> (182.0197, 46.516)
  arc A83 (182.1217, 46.414) -> (182.0197, 46.516) centre (182.0197, 46.414) ccw
  line L119 (182.1217, 46.414) -> (182.1217, 44.906)
  circle A84 centre (211.58, 45.04) radius 0.85
  arc A85 (164.6322, 42.264) -> (164.7342, 42.366) centre (164.6322, 42.366) ccw
  line L120 (164.6322, 42.264) -> (162.6322, 42.264)
  arc A86 (162.5302, 42.366) -> (162.6322, 42.264) centre (162.6322, 42.366) ccw
  line L121 (162.5302, 42.366) -> (162.5302, 43.874)
  arc A87 (162.6322, 43.976) -> (162.5302, 43.874) centre (162.6322, 43.874) ccw
  line L122 (162.6322, 43.976) -> (164.6322, 43.976)
  arc A88 (164.7342, 43.874) -> (164.6322, 43.976) centre (164.6322, 43.874) ccw
  line L123 (164.7342, 43.874) -> (164.7342, 42.366)
  arc A89 (182.0197, 42.264) -> (182.1217, 42.366) centre (182.0197, 42.366) ccw
  line L124 (182.0197, 42.264) -> (180.0197, 42.264)
  arc A90 (179.9177, 42.366) -> (180.0197, 42.264) centre (180.0197, 42.366) ccw
  line L125 (179.9177, 42.366) -> (179.9177, 43.874)
  arc A91 (180.0197, 43.976) -> (179.9177, 43.874) centre (180.0197, 43.874) ccw
  line L126 (180.0197, 43.976) -> (182.0197, 43.976)
  arc A92 (182.1217, 43.874) -> (182.0197, 43.976) centre (182.0197, 43.874) ccw
  line L127 (182.1217, 43.874) -> (182.1217, 42.366)
  circle A93 centre (129.53, 40.19) radius 1.3
  circle A94 centre (210.09, 40.19) radius 1.3
  arc A95 (164.6322, 39.724) -> (164.7342, 39.826) centre (164.6322, 39.826) ccw
  line L128 (164.6322, 39.724) -> (162.6322, 39.724)
  arc A96 (162.5302, 39.826) -> (162.6322, 39.724) centre (162.6322, 39.826) ccw
  line L129 (162.5302, 39.826) -> (162.5302, 41.334)
  arc A97 (162.6322, 41.436) -> (162.5302, 41.334) centre (162.6322, 41.334) ccw
  line L130 (162.6322, 41.436) -> (164.6322, 41.436)
  arc A98 (164.7342, 41.334) -> (164.6322, 41.436) centre (164.6322, 41.334) ccw
  line L131 (164.7342, 41.334) -> (164.7342, 39.826)
  arc A99 (182.0197, 39.724) -> (182.1217, 39.826) centre (182.0197, 39.826) ccw
  line L132 (182.0197, 39.724) -> (180.0197, 39.724)
  arc A100 (179.9177, 39.826) -> (180.0197, 39.724) centre (180.0197, 39.826) ccw
  line L133 (179.9177, 39.826) -> (179.9177, 41.334)
  arc A101 (180.0197, 41.436) -> (179.9177, 41.334) centre (180.0197, 41.334) ccw
  line L134 (180.0197, 41.436) -> (182.0197, 41.436)
  arc A102 (182.1217, 41.334) -> (182.0197, 41.436) centre (182.0197, 41.334) ccw
  line L135 (182.1217, 41.334) -> (182.1217, 39.826)
  line L136 (139.26, 40.74) -> (139.26, 38.54)
  line L137 (139.26, 38.54) -> (138.06, 38.54)
  line L138 (138.06, 38.54) -> (138.06, 40.74)
  line L139 (138.06, 40.74) -> (139.26, 40.74)
  line L140 (154.86, 40.74) -> (154.86, 38.54)
  line L141 (154.86, 38.54) -> (153.66, 38.54)
  line L142 (153.66, 38.54) -> (153.66, 40.74)
  line L143 (153.66, 40.74) -> (154.86, 40.74)
  arc A103 (164.6322, 37.184) -> (164.7342, 37.286) centre (164.6322, 37.286) ccw
  line L144 (164.6322, 37.184) -> (162.6322, 37.184)
  arc A104 (162.5302, 37.286) -> (162.6322, 37.184) centre (162.6322, 37.286) ccw
  line L145 (162.5302, 37.286) -> (162.5302, 38.794)
  arc A105 (162.6322, 38.896) -> (162.5302, 38.794) centre (162.6322, 38.794) ccw
  line L146 (162.6322, 38.896) -> (164.6322, 38.896)
  arc A106 (164.7342, 38.794) -> (164.6322, 38.896) centre (164.6322, 38.794) ccw
  line L147 (164.7342, 38.794) -> (164.7342, 37.286)
  arc A107 (182.0197, 37.184) -> (182.1217, 37.286) centre (182.0197, 37.286) ccw
  line L148 (182.0197, 37.184) -> (180.0197, 37.184)
  arc A108 (179.9177, 37.286) -> (180.0197, 37.184) centre (180.0197, 37.286) ccw
  line L149 (179.9177, 37.286) -> (179.9177, 38.794)
  arc A109 (180.0197, 38.896) -> (179.9177, 38.794) centre (180.0197, 38.794) ccw
  line L150 (180.0197, 38.896) -> (182.0197, 38.896)
  arc A110 (182.1217, 38.794) -> (182.0197, 38.896) centre (182.0197, 38.794) ccw
  line L151 (182.1217, 38.794) -> (182.1217, 37.286)
  circle A111 centre (129.53, 40.19) radius 7.0709
  circle A112 centre (129.53, 102.8) radius 8.2979
  circle A113 centre (210.09, 102.8) radius 9.4302
  circle A114 centre (213.2354, 37.5998) radius 5.7576
  constraint concentric A93 A111
  constraint concentric A3 A112
  constraint concentric A2 A113
extrude "Extrude5" add sketch "Sketch6" along normal blind 20.4 contours L4 L5 A2 L6 L7 A113 | A7 picked at (207.1072, 106.4281)